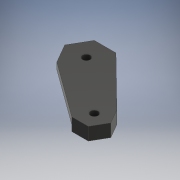
# Autodesk Inventor part: HA10
Saved by Autodesk Inventor 2017 (Build 210142000, 142)
## iProperties
Created: 2019-11-20
Part Number: HA10
Material: ABS Plastic
Document SubType Name: Modeling
Designer: Dell
Density: 1.06 g/cm^3
Appearance: Smooth - Black
Author: Dell
Autodesk Inventor part; units mm, degrees
ref_plane "YZ Plane" through (0, 0, 0) normal (1, 0, 0) x (0, 1, 0)
ref_plane "XZ Plane" through (0, 0, 0) normal (0, 1, 0) x (-1, 0, 0)
ref_plane "XY Plane" through (0, 0, 0) normal (0, 0, 1) x (1, 0, 0)
sketch "Sketch1" plane through (0, 0, 0) normal (0, 0, 1) x (1, 0, 0)
  circle A0 centre (0, 0) radius 12 construction
  line L0 (-51.9615, 0) -> (-25.9808, 45)
  line L1 (-25.9808, 45) -> (25.9808, 45)
  line L2 (25.9808, 45) -> (51.9615, 0)
  line L3 (51.9615, 0) -> (25.9808, -45)
  line L4 (25.9808, -45) -> (-25.9808, -45)
  line L5 (-25.9808, -45) -> (-51.9615, 0)
  dimension "d0" = 24
  dimension "d1" = 90
  constraints: 12 end point, 2 coincident, 1 centre point, 1 horizontal alignment, 13 other
  measures "d0" diameter of A0
  measures "d1" distance between parallel lines of L4 L1
extrude "Extrusion1" add sketch "Sketch1" along normal blind 40
sketch "Sketch2" plane through (0, 0, 0) normal (0, 0, -1) x (-1, 0, 0)
  line L0 (38.1051, 0) -> (19.0526, -33)
  line L1 (19.0526, -33) -> (-19.0526, -33)
  line L2 (-19.0526, -33) -> (-38.1051, 0)
  line L3 (-38.1051, 0) -> (-19.0526, 33)
  line L4 (-19.0526, 33) -> (19.0526, 33)
  line L5 (19.0526, 33) -> (38.1051, 0)
  circle A0 centre (0, 0) radius 12
  dimension "d4" = 24
  dimension "d5" = 66
  constraints: 12 end point, 2 coincident, 1 centre point, 1 horizontal alignment, 13 other
  measures "d4" diameter of A0
  measures "d5" distance between parallel lines of L1 L4
extrude "Extrusion2" cut sketch "Sketch2" against normal blind 13 contours L0 L1 L2 L3 L4 L5 | A0
sketch "Sketch3" plane through (0, 0, 40) normal (0, 0, 1) x (1, 0, 0)
  line L0 (-25.9808, -45) -> (25.9808, -45) projected
  line L1 (-25.9808, -45) -> (-199.0637, 81)
  line L2 (25.9808, 45) -> (-25.9808, 45) projected
  line L3 (25.9808, 45) -> (-130.9363, 199)
  line L4 (-51.9615, 0) -> (-25.9808, -45) projected
  line L5 (-25.9808, 45) -> (-51.9615, 0) projected
  line L6 (-130.9363, 199) -> (-96.8727, 140)
  line L7 (-96.8727, 140) -> (-130.9363, 81)
  line L8 (-130.9363, 81) -> (-199.0637, 81)
  line L9 (-199.0637, 81) -> (-233.1273, 140)
  line L10 (-233.1273, 140) -> (-199.0637, 199)
  line L11 (-199.0637, 199) -> (-130.9363, 199)
  point P0 (0, 0)
  point P1 (-165, 140)
  dimension "d9" = 165
  dimension "d21" = 140
  dimension "d22" = 118
  constraints: 16 end point, 1 horizontal, 13 other
  measures "d9" horizontal distance of point (0, 0) point (-165, 140)
  measures "d21" vertical distance of point (0, 0) point (-165, 140)
  measures "d22" distance between parallel lines of L8 L11
extrude "Extrusion3" add sketch "Sketch3" against normal blind 20.5
sketch "Sketch4" plane through (0, 0, 13) normal (0, 0, -1) x (-1, 0, 0)
  circle A0 centre (0, 0) radius 12
  dimension "d12" = 24
  constraints: 1 centre point, 1 coincident
  measures "d12" diameter of A0
extrude "Extrusion4" cut sketch "Sketch4" against normal through all
sketch "Sketch5" plane through (0, 0, 19.5) normal (0, 0, -1) x (-1, 0, 0)
  line L0 (199.0637, 199) -> (130.9363, 199) projected
  line L1 (201.9504, 140) -> (183.4752, 108)
  line L2 (183.4752, 108) -> (146.5248, 108)
  line L3 (146.5248, 108) -> (128.0496, 140)
  line L4 (128.0496, 140) -> (146.5248, 172)
  line L5 (146.5248, 172) -> (183.4752, 172)
  line L6 (183.4752, 172) -> (201.9504, 140)
  point P0 (0, 0)
  point P1 (165, 140)
  point P2 (165, 199)
  point P3 (233.1273, 140)
  dimension "d15" = 64
  constraints: 12 end point, 1 horizontal, 1 horizontal alignment, 1 midpoint, 1 vertical alignment, 13 other
  measures "d15" distance between parallel lines of L2 L5
extrude "Extrusion5" add sketch "Sketch5" along normal blind 13
sketch "Sketch6" plane through (0, 0, 6.5) normal (0, 0, -1) x (-1, 0, 0)
  circle A0 centre (165, 140) radius 12
  line L0 (183.4752, 172) -> (146.5248, 172) projected
  point P0 (0, 0)
  point P1 (201.9504, 140)
  point P2 (165, 172)
  dimension "d18" = 24
  constraints: 1 centre point, 1 horizontal alignment, 1 midpoint, 1 vertical alignment
  measures "d18" diameter of A0
extrude "Extrusion6" cut sketch "Sketch6" against normal through all
body "Solid1"
